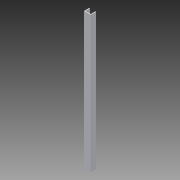
# Autodesk Inventor part: 26in C-Channel Right
Saved by Autodesk Inventor 2013 (Build 170138000, 138)
## iProperties
Created: 2013-01-08
Part Number: 26in C-Channel Right
Material: Aluminum 6061
Document SubType Name: Modeling
Designer: Naphat
Density: 1 g/cm^3
Author: Naphat
Autodesk Inventor part; units mm, degrees
ref_plane "YZ Plane" through (0, 0, 0) normal (1, 0, 0) x (0, 1, 0)
ref_plane "XZ Plane" through (0, 0, 0) normal (0, 1, 0) x (-1, 0, 0)
ref_plane "XY Plane" through (0, 0, 0) normal (0, 0, 1) x (1, 0, 0)
sketch "Sketch1" plane through (0, 0, 0) normal (0, 0, 1) x (1, 0, 0)
  line L0 (-16, 12.5) -> (-13, 12.5)
  line L1 (-13, 12.5) -> (-13, -9.5)
  line L2 (-13, -9.5) -> (13, -9.5)
  line L3 (13, -9.5) -> (13, 12.5)
  line L4 (13, 12.5) -> (16, 12.5)
  line L5 (16, 12.5) -> (16, -12.5)
  line L6 (16, -12.5) -> (-16, -12.5)
  line L7 (-16, -12.5) -> (-16, 12.5)
  point P0 (0, 0)
  dimension "d0" = 3
  dimension "d2" = 3
  dimension "d3" = 25
  dimension "d4" = 32
  dimension "d5" = 16
  dimension "d7" = 12.5
  dimension "d8" = 3
  dimension "d74" = 25
  constraints: 16 end point, 5 parallel, 1 collinear, 1 horizontal, 1 perpendicular
  measures "d0" distance of L0.start L0.end
  measures "d2" distance of L3.end L4.end
  measures "d3" distance of L6.end L0.start
  measures "d4" distance of L5.end L6.end
  measures "d5" distance from line of point (0, 0) L7
  measures "d7" distance from line of L6 point (0, 0)
  measures "d8" distance between parallel lines of L6 L2
  measures "d74" distance between parallel lines of L6 L4
extrude "Extrusion1" add sketch "Sketch1" against normal blind 660.4
sketch "Sketch6" plane through (-16, -12.5, 0) normal (-1, 0, 0) x (0, 0, 1)
  circle A0 centre (-37.4708, 12.3) radius 3.175
  circle A1 centre (-177.8, 12.3) radius 3.175
  circle A2 centre (-340.3166, 12.3) radius 3.175
  circle A3 centre (-644.4, 15.5) radius 3.175
  line L0 (0, 25) -> (-660.4, 25) projected
  line L1 (0, 3) -> (-660.4, 3) projected
  line L2 (-660.4, 0) -> (-660.4, 25) projected
  circle A4 centre (-16, 15.5) radius 3.175
  line L3 (0, 0) -> (0, 25) projected
  point P0 (0, 12.5)
  dimension "d89" = 6.35
  dimension "d92" = 16
  dimension "d93" = 6.35
  dimension "d94" = 16
  dimension "d103" = 12.5
  constraints: 5 centre point, 1 horizontal alignment
  measures "d89" diameter of A3
  measures "d92" distance from line of L2 A3.centre
  measures "d93" diameter of A4
  measures "d94" distance from line of A4.centre L3
  measures "d103" distance from line of A3.centre L1
hole "Hole3" at (-16, 3, -644.4) at (-16, 3, -16) direction (1, 0, 0) diameter 6.35 depth 3 tip angle 118
equation "\"d2\" = d0"
equation "\"d5\" = 0.5 * d4"
equation "\"d7\" = 0.5 * d3"
equation "\"d8\" = d0"
equation "\"d74\" = d3"
body "Solid1"
